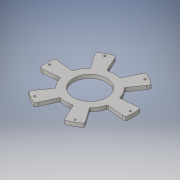
# Autodesk Inventor part: Arm Mount
Saved by Autodesk Inventor 2016 (Build 200138000, 138)
## iProperties
Created: 2016-04-16
Part Number: Arm Mount
Material: Generic
Document SubType Name: Modeling
Designer: rmarkowi
Density: 1 g/cm^3
Appearance: Default
Author: rmarkowi
Autodesk Inventor part; units mm, degrees
ref_plane "YZ Plane" through (0, 0, 0) normal (1, 0, 0) x (0, 1, 0)
ref_plane "XZ Plane" through (0, 0, 0) normal (0, 1, 0) x (-1, 0, 0)
ref_plane "XY Plane" through (0, 0, 0) normal (0, 0, 1) x (1, 0, 0)
sketch "Sketch1" plane through (0, 0, 0) normal (0, 1, 0) x (-1, 0, 0)
  circle A0 centre (0, 0) radius 57.15
  circle A1 centre (0, 0) radius 137.541 construction
  circle A2 centre (137.541, 0) radius 3.175
  circle A3 centre (68.7705, 119.114) radius 3.175
  circle A4 centre (-68.7705, 119.114) radius 3.175
  circle A5 centre (-137.541, 0) radius 3.175
  circle A6 centre (-68.7705, -119.114) radius 3.175
  circle A7 centre (68.7705, -119.114) radius 3.175
  arc A8 (89.500903, 104.437134) -> (45.69476, 129.728623) centre (68.7705, 119.114) ccw
  line L0 (45.69476, 129.728623) -> (23.666851, 81.840883)
  line L1 (89.500903, 104.437134) -> (59.042858, 61.416536)
  arc A9 (59.042858, 61.416536) -> (59.351412, 57.37519) centre (61.634159, 59.581928) ccw
  arc A10 (20.012666, 80.087425) -> (23.666851, 81.840883) centre (20.782384, 83.167711) ccw
  line L2 (-45.69476, 129.728623) -> (-23.666851, 81.840883)
  arc A11 (-23.666851, 81.840883) -> (-20.012666, 80.087425) centre (-20.782384, 83.167711) ccw
  line L3 (-89.500903, 104.437134) -> (-59.042858, 61.416536)
  arc A12 (-59.351412, 57.37519) -> (-59.042858, 61.416536) centre (-61.634159, 59.581928) ccw
  arc A13 (-45.69476, 129.728623) -> (-89.500903, 104.437134) centre (-68.7705, 119.114) ccw
  line L4 (-135.195663, 25.291489) -> (-82.709709, 20.424347)
  arc A14 (-82.709709, 20.424347) -> (-79.364078, 22.712236) centre (-82.416542, 23.585783) ccw
  line L5 (-135.195663, -25.291489) -> (-82.709709, -20.424347)
  arc A15 (-79.364078, -22.712236) -> (-82.709709, -20.424347) centre (-82.416542, -23.585783) ccw
  arc A16 (-135.195663, 25.291489) -> (-135.195663, -25.291489) centre (-137.541, 0) ccw
  line L6 (-89.500903, -104.437134) -> (-59.042858, -61.416536)
  arc A17 (-59.042858, -61.416536) -> (-59.351412, -57.37519) centre (-61.634159, -59.581928) ccw
  line L7 (-45.69476, -129.728623) -> (-23.666851, -81.840883)
  arc A18 (-20.012666, -80.087425) -> (-23.666851, -81.840883) centre (-20.782384, -83.167711) ccw
  arc A19 (-89.500903, -104.437134) -> (-45.69476, -129.728623) centre (-68.7705, -119.114) ccw
  line L8 (45.69476, -129.728623) -> (23.666851, -81.840883)
  arc A20 (23.666851, -81.840883) -> (20.012666, -80.087425) centre (20.782384, -83.167711) ccw
  line L9 (89.500903, -104.437134) -> (59.042858, -61.416536)
  arc A21 (59.351412, -57.37519) -> (59.042858, -61.416536) centre (61.634159, -59.581928) ccw
  arc A22 (45.69476, -129.728623) -> (89.500903, -104.437134) centre (68.7705, -119.114) ccw
  line L10 (135.195663, -25.291489) -> (82.709709, -20.424347)
  arc A23 (82.709709, -20.424347) -> (79.364078, -22.712236) centre (82.416542, -23.585783) ccw
  line L11 (135.195663, 25.291489) -> (82.709709, 20.424347)
  arc A24 (79.364078, 22.712236) -> (82.709709, 20.424347) centre (82.416542, 23.585783) ccw
  arc A25 (135.195663, -25.291489) -> (135.195663, 25.291489) centre (137.541, 0) ccw
  arc A26 (79.364078, 22.712236) -> (59.351412, 57.37519) centre (0, 0) ccw
  arc A27 (59.351412, -57.37519) -> (79.364078, -22.712236) centre (0, 0) ccw
  arc A28 (-20.012666, -80.087425) -> (20.012666, -80.087425) centre (0, 0) ccw
  arc A29 (-79.364078, -22.712236) -> (-59.351412, -57.37519) centre (0, 0) ccw
  arc A30 (20.012666, 80.087425) -> (-20.012666, 80.087425) centre (0, 0) ccw
  arc A31 (-59.351412, 57.37519) -> (-79.364078, 22.712236) centre (0, 0) ccw
  arc A32 (45.69476, -129.728623) -> (52.30591, -138.455078) centre (68.7705, -119.114) ccw
  arc A33 (93.752659, -114.525786) -> (89.500903, -104.437134) centre (68.7705, -119.114) ccw
  arc A34 (146.05857, 23.929292) -> (135.195663, 25.291489) centre (137.541, 0) ccw
  arc A35 (135.195663, -25.291489) -> (146.05857, -23.929292) centre (137.541, 0) ccw
  arc A36 (52.30591, 138.455078) -> (45.69476, 129.728623) centre (68.7705, 119.114) ccw
  arc A37 (89.500903, 104.437134) -> (93.752659, 114.525786) centre (68.7705, 119.114) ccw
  arc A38 (-93.752659, 114.525786) -> (-89.500903, 104.437134) centre (-68.7705, 119.114) ccw
  arc A39 (-45.69476, 129.728623) -> (-52.30591, 138.455078) centre (-68.7705, 119.114) ccw
  arc A40 (-146.05857, -23.929292) -> (-135.195663, -25.291489) centre (-137.541, 0) ccw
  arc A41 (-135.195663, 25.291489) -> (-146.05857, 23.929292) centre (-137.541, 0) ccw
  arc A42 (-52.30591, -138.455078) -> (-45.69476, -129.728623) centre (-68.7705, -119.114) ccw
  arc A43 (-89.500903, -104.437134) -> (-93.752659, -114.525786) centre (-68.7705, -119.114) ccw
  point P0 (-52.30591, -138.455078)
  point P1 (-93.752659, -114.525786)
  dimension "d0" = 114.3
  dimension "d2" = 275.082
  dimension "d3" = 6.35
  dimension "d6" = 360
  dimension "d8" = 50.8
  dimension "d9" = 6.35
  dimension "d10" = 6.35
  dimension "d13" = 360
  dimension "d20" = 360
  constraints: 83 point on circle, 44 centre point, 24 end point, 4 coincident, 4 tangent, 141 other
  measures "d0" diameter of A0
  measures "d2" diameter of A1
  measures "d3" diameter of A2
  measures "d8" diameter of A8
  measures "d9" diameter of A9
  measures "d10" diameter of A10
extrude "Extrusion1" add sketch "Sketch1" along normal blind 12.7
sketch "Sketch2" plane through (0, 12.7, 0) normal (0, 1, 0) x (1, 0, 0)
  circle A0 centre (0, 0) radius 148.0058
  circle A1 centre (0, 0) radius 162.941
  dimension "d26" = 296.0116
  constraints: 2 centre point, 1 coincident
  measures "d26" diameter of A0
extrude "Extrusion3" cut sketch "Sketch2" against normal through all
body "Solid1"
